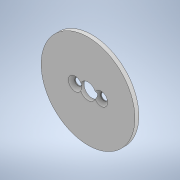
# Autodesk Inventor part: SlitDiscSupport1
Saved by Autodesk Inventor 2022 (Build 260153000, 153)
## iProperties
Created: 2024-08-21
Part Number: SlitDiscSupport1
Material: 一般
Document SubType Name: Modeling
Designer: yamashita1
Density: 1 g/cm^3
Appearance: 既定
Author: yamashita1
Autodesk Inventor part; units mm, degrees
ref_plane "YZ Plane" through (0, 0, 0) normal (1, 0, 0) x (0, 1, 0)
ref_plane "XZ Plane" through (0, 0, 0) normal (0, 1, 0) x (-1, 0, 0)
ref_plane "XY Plane" through (0, 0, 0) normal (0, 0, 1) x (1, 0, 0)
sketch "スケッチ1" plane through (0, 0, 0) normal (0, 0, 1) x (1, 0, 0)
  circle A0 centre (0, 0) radius 23.5
  circle A1 centre (0, 0) radius 4
  dimension "d0" = 47
  dimension "d1" = 8
  constraints: 2 centre point, 2 coincident
  measures "d0" diameter of A0
  measures "d1" diameter of A1
extrude "押し出し1" add sketch "スケッチ1" along normal blind 2
sketch "スケッチ2" plane through (0, 0, 2) normal (0, 0, 1) x (1, 0, 0)
  circle A0 centre (0, 0) radius 6.5 construction
  circle A1 centre (-6.5, 0) radius 1.75
  circle A2 centre (6.5, 0) radius 1.75
  dimension "d4" = 13
  dimension "d5" = 3.5
  constraints: 3 centre point, 2 horizontal alignment, 2 point on circle, 1 coincident, 1 equal radius
  measures "d4" diameter of A0
  measures "d5" diameter of A1
extrude "押し出し2" cut sketch "スケッチ2" against normal blind 2
chamfer "面取り1" distance 1.6 angle 45 2 edges at (-8.25, 0, 2) (4.75, 0, 2)
